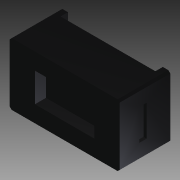
# Autodesk Inventor part: AS11CHright1
Saved by Autodesk Inventor 2011 SP1 (Build 150282100, 282)
## iProperties
Created: 2018-06-01
Part Number: AS11CHright1
Catalog Web Link: www.cadenas.de
Description: AS - Series - Body 1 for Poles 1 - Right Angle-
Vendor: NKKSWITCHES
Document SubType Name: Modeling
Designer: psAdmin
Manufacturer: NKKSWITCHES
Mass: 0.153997 g
Surface Area: 2.19857 cm^2
Volume: 0.153997 cm^3
Density: 1 g/cm^3
Category: PARTsolutions
Company: NKKSWITCHES
Title: AS11CHright1
Author: Cadenas PARTsolutions
PSOL_IDENT_0: {$CADENAS_DATA\23d-libs\nkkswitches\slides\as\parts\as_body_right1.prj},227 {VTYP=3D},{NB=AS11CHrigh
PSOL_IDENT_1: t1},{LINA=AS11CHright1},{NN=AS - Series - Body 1 for Poles 1 - Right Angle},{DATE=11.10.2017 10:53:5
PSOL_IDENT_2: 0},{GEOMDATE=09.12.2008 09:45:00},{VERSION=},{LINEID=10},{LINESUBID=-1},{WBVAR=PLS,CRCTS,ACTU,TRMNLS
PSOL_IDENT_3: }  {NB=AS11CHright1},{LINA=AS11CHright1},{KT=DUMMY},{PN=AS11CH},{SRS=AS},{PLS=1},{CRCTS=1},{ACTU=C},
PSOL_IDENT_4: {TRMNLS=H},{CCLR=0.00,0.00,0.00,0.00},{CRCTSALG=  '1', '1 - ON/NONE/OFF','2', '2 - ON/NONE/ON', '3',
PSOL_IDENT_5: '3 - ON/OFF/ON' }
NN: AS - Series - Body 1 for Poles 1 - Right Angle
NB: AS11CHright1
NBSYN: $PN.right1
LINA: AS11CHright1
PN: AS11CH
SRS: AS
PLS: 1 - SPST/SPDT
CRCTS: 1 - ON/NONE/OFF
ACTU: C - .150"(3,8mm)Long
TRMNLS: H - Right Angle with Bracket
SUPPLIER: NKKSWITCHES
ARTICLENO: AS11CHright1
BOMINFO: AS11CHright1
CREATOR: CADENAS GmbH
Autodesk Inventor part; units mm, degrees
sketch "Sketch_1" plane through (0, 0, 0) normal (0, 0, 1) x (1, 0, 0)
  line L0 (-4.4958, -2.3876) -> (-4.3434, -2.54)
  line L1 (-4.3434, -2.54) -> (4.3434, -2.54)
  line L2 (4.3434, -2.54) -> (4.4958, -2.3876)
  line L3 (4.4958, -2.3876) -> (4.4958, 2.3876)
  line L4 (4.4958, 2.3876) -> (4.3434, 2.54)
  line L5 (4.3434, 2.54) -> (-4.3434, 2.54)
  line L6 (-4.3434, 2.54) -> (-4.4958, 2.3876)
  line L7 (-4.4958, 2.3876) -> (-4.4958, -2.3876)
  constraints: 16 end point
extrude "Extrusion1" add sketch "Sketch_1" along normal blind 4.1529
sketch "Sketch_5" plane through (0, 0, 4.1529) normal (0, 0, 1) x (1, 0, 0)
  line L0 (-2.4384, 1.1938) -> (-2.4384, -1.1938)
  line L1 (-2.4384, -1.1938) -> (2.4384, -1.1938)
  line L2 (2.4384, -1.1938) -> (2.4384, 1.1938)
  line L3 (2.4384, 1.1938) -> (-2.4384, 1.1938)
  constraints: 8 end point
extrude "Extrusion2" cut sketch "Sketch_5" against normal blind 0.9144
sketch "Sketch_4" plane through (4.4958, 0, 0) normal (1, 0, 0) x (0, 0, -1)
  line L0 (-2.54, 1.27) -> (-2.54, -1.27)
  line L1 (-2.54, -1.27) -> (-1.9304, -1.27)
  line L2 (-1.9304, -1.27) -> (-1.9304, 1.27)
  line L3 (-1.9304, 1.27) -> (-2.54, 1.27)
  constraints: 8 end point
extrude "Extrusion3" cut sketch "Sketch_4" against normal blind 0.254
sketch "Sketch_6" plane through (-4.4958, 0, 0) normal (1, 0, 0) x (0, 0, -1)
  line L0 (-2.54, 1.27) -> (-2.54, -1.27)
  line L1 (-2.54, -1.27) -> (-1.9304, -1.27)
  line L2 (-1.9304, -1.27) -> (-1.9304, 1.27)
  line L3 (-1.9304, 1.27) -> (-2.54, 1.27)
  constraints: 8 end point
extrude "Extrusion4" cut sketch "Sketch_6" along normal blind 0.254
sketch "Sketch_2" plane through (0, 0, 0) normal (0, 0, 1) x (1, 0, 0)
  line L0 (-3.8862, 2.54) -> (-3.8862, -2.54)
  line L1 (-3.8862, -2.54) -> (3.8862, -2.54)
  line L2 (3.8862, -2.54) -> (3.8862, 2.54)
  line L3 (3.8862, 2.54) -> (-3.8862, 2.54)
  constraints: 8 end point
extrude "Extrusion5" cut sketch "Sketch_2" along normal blind 0.6096
ref_plane "actu_a_right_XY" through (-0.0508, 0, 3.2385) normal (0, 0, -1) x (1, 0, 0)
ref_plane "actu_a_right_YZ" through (-0.0508, 0, 3.2385) normal (1, 0, 0) x (0, -1, 0)
ref_plane "actu_a_right_ZX" through (-0.0508, 0, 3.2385) normal (0, -1, 0) x (0, 0, -1)
ref_plane "body12_right_XY" through (0, 0, 0.6096) normal (0, 0, 1) x (1, 0, 0)
ref_plane "body12_right_YZ" through (0, 0, 0.6096) normal (1, 0, 0) x (0, 1, 0)
ref_plane "body12_right_ZX" through (0, 0, 0.6096) normal (0, 1, 0) x (0, 0, 1)
body "Solid1"
